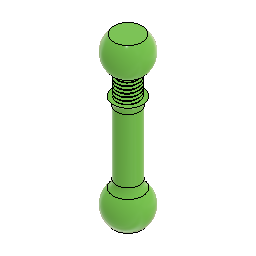
ball joint v2_ball+thread+2cm v3 (Autodesk Fusion 360 design; units mm, degrees)
Autodesk Fusion 360 part; units mm, degrees
sketch "Skizze1" plane through (0, 0, 0) normal (0, 1, 0) x (1, 0, 0)
  line L0 (0, 0) -> (15, 0)
  line L1 (15, 0) -> (15, -10)
  line L2 (15, -10) -> (0, -10)
  line L3 (0, -10) -> (0, 0)
  line L4 (0, 0) -> (0, -48.75)
  circle A0 centre (0, -22.5) radius 11.25
  line L5 (0, -48.75) -> (7.5984, -48.75)
  line L6 (7.5984, -48.75) -> (7.5984, -41.25)
  line L7 (7.5984, -41.25) -> (0, -41.25)
  line L8 (7.5984, -41.25) -> (9.4734, -41.25)
  line L9 (9.4734, -41.25) -> (9.4734, -39.25)
  spline S0 degree 2 poles (9.4734, -39.25) (5, -35) (6.25, -31.8541) knots 0 0 0 0.889763 0.889763 0.889763 weights 1 3 1
  line L10 (0, -14.25) -> (7.6485, -14.25)
  line L11 (13.7326, -10) -> (13.7326, -21.25)
  line L12 (13.7326, -21.25) -> (11.1803, -21.25)
  line L13 (13.7326, -21.25) -> (13.7326, -23.125)
  line L14 (13.7326, -23.125) -> (11.2326, -23.125)
  line L15 (13.7326, -12.875) -> (15.2326, -12.875)
  line L16 (17.7326, -15.375) -> (17.7326, -25.625)
  line L17 (15.2326, -28.125) -> (10.5734, -28.125)
  arc A1 (10.1235, -27.4069) -> (10.5734, -28.125) centre (10.5734, -27.625) ccw
  arc A2 (15.2326, -28.125) -> (17.7326, -25.625) centre (15.2326, -25.625) ccw
  arc A3 (17.7326, -15.375) -> (15.2326, -12.875) centre (15.2326, -15.375) ccw
  line L18 (0, -22.5) -> (11.25, -22.5) construction
  line L19 (10.5734, -27.625) -> (10.0734, -27.625) construction
  line L20 (10.0734, -27.625) -> (10.0734, -56.869) construction
  point P0 (0, -11.25)
  point P1 (0, -33.75)
  dimension "d1" = 15
  dimension "d2" = 10
  dimension "d3" = 0
  dimension "d4" = 0
  dimension "d5" = 0
  dimension "d6" = 0
  dimension "d7" = 0
  dimension "d8" = 0
  dimension "d9" = 0
  dimension "d10" = 0
  dimension "d11" = 0
  dimension "d12" = 0.5
  dimension "d13" = 0
  dimension "d14" = 0
  dimension "d15" = 0
  dimension "d16" = 0
  dimension "d17" = 0
  dimension "d18" = 0
  dimension "d19" = 0
  dimension "d20" = 0.6
  dimension "d21" = 0
  dimension "d22" = 4
  constraint horizontal L0
  constraint vertical L1
  constraint horizontal L2
  constraint vertical L3
  constraint coincident L0.start L3.end
  constraint perpendicular L0 L4
  constraint coincident L4 A0.centre
  constraint coincident A0 P0
  constraint coincident L4 P0
  constraint perpendicular L4 L5
  constraint perpendicular L5 L6
  constraint coincident L4 L7.end
  constraint perpendicular L4 L7
  constraint perpendicular L6 L8
  constraint perpendicular L8 L9
  constraint coincident A0 S0.end
  constraint coincident A0 P1
  constraint coincident L4 P1
  constraint coincident L4 L10.start
  constraint coincident A0 L10.end
  constraint perpendicular L4 L10
  constraint coincident L2 L11.start
  constraint perpendicular L2 L11
  constraint coincident A0 L12.end
  constraint perpendicular L11 L12
  constraint perpendicular L12 L13
  constraint perpendicular L13 L14
  constraint coincident L11 L15.start
  constraint perpendicular L11 L15
  constraint perpendicular L15 L16
  constraint perpendicular L16 L17
  constraint tangent L17 A1
  constraint coincident A0 A1.start
  constraint tangent L17 A2
  constraint tangent L16 A2
  constraint tangent L15 A3
  constraint tangent L16 A3
  constraint coincident A0.centre L18.start
  constraint perpendicular L4 L18
  constraint coincident A0 L14.end
  constraint coincident A0 L18.end
  constraint coincident A1.centre L19.start
  constraint coincident A1 L19.end
  constraint horizontal L19
  constraint tangent A0 A1
  constraint tangent A1 L20
  measures "d1" distance of L0.start L0.end
  measures "d2" distance of L0.start L2.end
  measures "d4" distance of L2.end P0
  measures "d5" distance of L5.end L6.end
  measures "d6" distance of L6.end L8.end
  measures "d7" distance of L8.end L9.end
  measures "d9" distance of L7 P1
  measures "d11" distance of L12 L14
  measures "d12" radius of A1
  measures "d18" distance of L13.end L14.end
  measures "d19" distance of L2 L15
  measures "d20" distance of L9 L20
  measures "d21" distance of L14 L17
  measures "d22" distance of L11 L16
revolve "Drehen1" add sketch "Skizze1" angle 360 about axis through (0, 0, 0) along (0, 0, 1) contours L4 A0 L10 | L4 A0 L7 L8 L9 S0 picked at (0.5502, -27.2094) makes body 1
sketch "Skizze2" plane through (0, 0, 0) normal (1, 0, 0) x (0, 1, 0)
  line L0 (7.6485, 14.25) -> (-7.6485, 14.25)
  line L1 (9.4734, 41.25) -> (-9.4734, 41.25)
  arc A0 (-6.25, 31.8541) -> (-7.6485, 14.25) centre (0, 22.5) ccw
  arc A1 (7.6485, 14.25) -> (6.25, 31.8541) centre (0, 22.5) ccw
  spline S0 degree 3 poles (9.4734, 39.25) (7.684, 37.55) (7.2201, 37.0637) (6.3323, 36.0999) (6.0974, 35.7971) (5.75, 35.2505) (5.6493, 35.0195) (5.5531, 34.5777) (5.5392, 34.3776) (5.5907, 33.8312) (5.6556, 33.4978) (5.9698, 32.5819) (6.0806, 32.2805) (6.25, 31.8541) knots 0 0 0 0 0.177953 0.177953 0.355905 0.355905 0.533858 0.533858 0.669964 0.669964 0.829466 0.829466 0.889763 0.889763 0.889763 0.889763
  spline S1 degree 3 poles (-9.4734, 39.25) (-7.684, 37.55) (-7.2201, 37.0637) (-6.3323, 36.0999) (-6.0974, 35.7971) (-5.75, 35.2505) (-5.6493, 35.0195) (-5.5531, 34.5777) (-5.5392, 34.3776) (-5.5907, 33.8312) (-5.6556, 33.4978) (-5.9698, 32.5819) (-6.0806, 32.2805) (-6.25, 31.8541) knots 0 0 0 0 0.177953 0.177953 0.355905 0.355905 0.533858 0.533858 0.669964 0.669964 0.829466 0.829466 0.889763 0.889763 0.889763 0.889763
  line L2 (9.4734, 39.25) -> (9.4734, 41.25)
  line L3 (-9.4734, 39.25) -> (-9.4734, 41.25)
ref_plane "Arbeitsebene1" through (0, 0, 31.8541) normal (0, 0, 1) x (1, 0, 0)
split "Teilen1" by plane through (0, 0, 31.8541) normal (0, 0, 1) bodies 1 makes body 2 at (6.4033, -1.2945, 36.3114)
delete_body "Körper entfernen1" bodies 2
extrude "Extrusion1" add 1 faces at (0.1138, -0.2899, 31.8541) along direction (0, 0, 1) blind 40 separate body on bodies 1 makes body 3
copy_body "Körper kopieren/einfügen1" bodies 1 makes body 4
move_body "Verschieben1" bodies 4 to x (1, 0, 0) y (0, 1, 0) z (0, 0, 1) at (0, -40, 0)
move_body "Ausrichten1" bodies 4 to x (1, 0, 0) y (0, -1, 0) z (0, 0, -1) at (0, -40, 103.7083)
combine "Kombinieren1" operation add target body 1 tool bodies 3 4
fillet "Abrundung1" radius 6 2 edges at (-5.827, -2.2601, 31.8541) (-5.827, -2.2601, 71.8541) on bodies 1
sketch "Skizze3" plane through (0, 0, 0) normal (1, 0, 0) x (0, 1, 0)
  line L0 (-7.9891, 73.2877) -> (7.9891, 73.2877)
ref_plane "Arbeitsebene2" through (0, 0, 73.2877) normal (0, 0, 1) x (-1, 0, 0)
split "Teilen2" by plane through (0, 0, 73.2877) normal (0, 0, 1) bodies 1 makes body 5 at (8.3516, 7.5198, 80.6934)
sketch "Skizze4" plane through (0, 0, 73.2877) normal (0, 0, 1) x (-1, 0, 0)
  circle A0 centre (0, 0) radius 7.9891
  circle A1 centre (0, 0) radius 5
  dimension "d29" = 10
  constraint coincident A0.centre A1.centre
  measures "d29" diameter of A1
extrude "Extrusion2" add sketch "Skizze4" along normal blind 10 contours A1 bodies 1
thread "Gewinde1" "ISO Metric profile 12.0 M12x1.75 6g" major diameter 11.8335 minor diameter 9.8365 pitch 1.75 angle 60 modelled right hand crest width 0.2518 on face at (-4.9938, 0.2492, 79.9543) crest through (-5.9168, 0, 72.8502) on bodies 1
sketch "Skizze5" plane through (0, 0, 73.2877) normal (0, 0, -1) x (1, 0, 0)
  circle A0 centre (0, 0) radius 7.9891
hole "Bohrung1" at (0, 0, 73.2877) direction (0, 0, 1) diameter 10.274 depth 11 tip angle 180 bodies 5
thread "Gewinde2" "ISO Metric profile 12.0 M12x1.75 6H" major diameter 12.2265 minor diameter 10.2735 pitch 1.75 angle 60 modelled right hand crest width 0.4769 on face at (0.2561, 5.1306, 76.9543) crest through (-5.1368, 0, 73.7252) on bodies 5
move_body "Move2" bodies 1 to x (1, 0, 0) y (0, 1, 0) z (0, 0, 1) at (0, 0, -13)
equation "d1 = 25 mm * 0.6"
equation "d3 = base * 18 / 12"
equation "d4 = base * 1 / 12"
equation "d5 = base * 6 / 12"
equation "d6 = base * 1.5 / 12"
equation "d7 = base * 1.6 / 12"
equation "d8 = base * 5 / 12"
equation "d9 = base * 6 / 12"
equation "d10 = base * 2.4 / 12"
equation "d11 = base * 1.5 / 12"
equation "d13 = base * 2 / 12"
equation "d14 = base * 2 / 12"
equation "d15 = base * 4 / 12"
equation "d16 = base * 1 / 12"
equation "d17 = base * 8 / 12"
equation "d18 = base * 2 / 12"
equation "d19 = ( base * 1.5 / 12 ) + 1 mm"
equation "d21 = base * 4 / 12"
